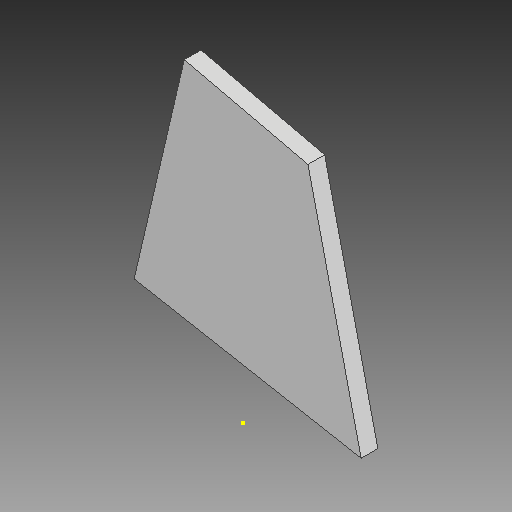
# Autodesk Inventor part: Seitenverkleidung
Saved by Autodesk Inventor 2021 (Build 250183000, 183)
## iProperties
Created: 2021-10-11
Part Number: Seitenverkleidung
Material: Generisch
Document SubType Name: Modeling
Designer: lukas
Density: 1 g/cm^3
Appearance: Vorgabe
Stock Number: Seitenverkleidung
Author: lukas
Autodesk Inventor part; units mm, degrees
ref_plane "YZ Plane" through (0, 0, 0) normal (1, 0, 0) x (0, 1, 0)
ref_plane "XZ Plane" through (0, 0, 0) normal (0, 1, 0) x (-1, 0, 0)
ref_plane "XY Plane" through (0, 0, 0) normal (0, 0, 1) x (1, 0, 0)
sketch "Skizze5" plane through (0, 0, 0) normal (0, 0, 1) x (1, 0, 0)
  line L0 (-515.9615, 0) -> (494.3584, 0) projected
  line L1 (0, -1109.8805) -> (0, 1119.7281) projected
  line L2 (0, 801.2126) -> (-371.6301, -791.365)
  line L3 (0, 801.2126) -> (350.027, -698.7874)
  line L4 (-87.4769, 426.3407) -> (97.5522, 383.1639)
  line L5 (97.5522, 383.1639) -> (177.0884, 42.3208)
  line L6 (-87.4769, 426.3407) -> (-162.4681, 104.9743)
  line L7 (-162.4681, 104.9743) -> (177.0884, 42.3208)
  point P0 (0, 0)
  point P1 (0, 401.2126)
  point P2 (-162.4681, 104.9743)
  point P3 (177.0884, 42.3208)
  dimension "d58" = 26.27
  dimension "d59" = 1500
  dimension "d60" = 400
  dimension "d63" = 190
  dimension "d64" = 330
  dimension "d65" = 350
  dimension "d66" = 0
  dimension "d67" = 0
  dimension "d68" = 90
  constraints: 12 end point, 4 point on line, 1 other
  measures "d58" angle of L3 L2
  measures "d59" vertical distance of L3.end L2.start
  measures "d60" distance of L2.start point (0, 401.213)
  measures "d63" distance of L4.start L4.end
  measures "d64" distance of L4.start L6.end
  measures "d65" distance of L4.end L5.end
  measures "d66" distance between parallel lines of L2 L6
  measures "d67" distance between parallel lines of L3 L5
  measures "d68" angle of L4 L2
extrude "Extrusion4" add sketch "Skizze5" along normal blind 25 contours L2 L4 L1 L7 | L1 L4 L3 L7
sketch "Skizze6" plane through (0, 0, 25) normal (0, 0, 1) x (1, 0, 0)
  point P0 (0, 0)
